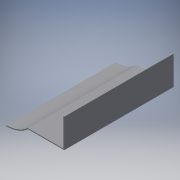
# Autodesk Inventor part: Part4
Saved by Autodesk Inventor 2016 (Build 200138000, 138)
## iProperties
Created: 2016-09-04
Part Number: Part4
Material: Aluminum 6061
Document SubType Name: Modeling
Designer: gus
Density: 2.7 g/cm^3
Appearance: Aluminum - Flat
Author: gus
Autodesk Inventor part; units mm, degrees
ref_plane "YZ Plane" through (0, 0, 0) normal (1, 0, 0) x (0, 1, 0)
ref_plane "XZ Plane" through (0, 0, 0) normal (0, 1, 0) x (-1, 0, 0)
ref_plane "XY Plane" through (0, 0, 0) normal (0, 0, 1) x (1, 0, 0)
sketch "Sketch1" plane through (0, 0, 0) normal (0, 0, 1) x (1, 0, 0)
  arc A0 (0, 0) -> (179.4192, 91.0867) centre (0, 222.25) ccw
  line L0 (0, 0) -> (177.8, 0) construction
  line L1 (179.4192, 91.0867) -> (306.4192, 91.0867)
  line L2 (306.4192, 91.0867) -> (306.4192, 243.4867)
  line L3 (303.2442, 94.2617) -> (303.2442, 243.4867)
  arc A1 (0, 3.175) -> (177.8, 94.2617) centre (0, 222.25) ccw
  line L4 (303.2442, 94.2617) -> (177.8, 94.2617)
  line L5 (0, 3.175) -> (0, 0)
  line L6 (303.2442, 243.4867) -> (306.4192, 243.4867)
  dimension "d0" = 222.25
  dimension "d2" = 152.4
  dimension "d3" = 127
  dimension "d6" = 3.175
  dimension "d7" = 3.175
  dimension "d8" = 3.175
  dimension "d9" = 3.175
  dimension "d12" = 177.8
  dimension "d13" = 177.8
  constraints: 14 end point, 4 horizontal, 4 point on circle, 2 centre point, 1 concentric, 1 perpendicular, 1 tangent
  measures "d0" radius of A0
  measures "d2" distance of L1.end L2.end
  measures "d3" distance of L1.start L1.end
  measures "d6" distance between parallel lines of L2 L3
  measures "d7" radial gap between concentric circles of A0 A1
  measures "d8" distance between parallel lines of L1 L4
  measures "d9" distance of L5.start L0.start
  measures "d12" distance of L0.start L0.end
  measures "d13" horizontal distance of L0.start L4.end
extrude "Extrusion1" add sketch "Sketch1" against normal blind 384.175
body "Solid1"
